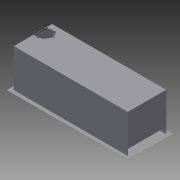
# Autodesk Inventor part: Restivo_Drawing
Saved by Autodesk Inventor 2013 SP2 (Build 170200200, 200)
## iProperties
Created: 2014-01-21
Part Number: Restivo_Drawing
Material: Generic
Document SubType Name: Modeling
Designer: mcgratta
Density: 1 g/cm^3
Author: mcgratta
Autodesk Inventor part; units mm, degrees
ref_plane "YZ Plane" through (0, 0, 0) normal (1, 0, 0) x (0, 1, 0)
ref_plane "XZ Plane" through (0, 0, 0) normal (0, 1, 0) x (-1, 0, 0)
ref_plane "XY Plane" through (0, 0, 0) normal (0, 0, 1) x (1, 0, 0)
sketch "Sketch1" plane through (0, 0, 0) normal (0, 1, 0) x (-1, 0, 0)
  line L0 (300, 300) -> (-9300, 300)
  line L1 (-9300, 300) -> (-9300, -3300)
  line L2 (-9300, -3300) -> (300, -3300)
  line L3 (300, -3300) -> (300, 300)
  point P0 (0, 0)
  dimension "d0" = 3600
  dimension "d2" = 9600
  dimension "d3" = 300
  dimension "d4" = 300
  constraints: 8 end point, 2 parallel, 1 horizontal, 1 perpendicular
  measures "d0" distance of L2.end L0.start
  measures "d2" distance between parallel lines of L1 L3
  measures "d3" distance from line of point (0, 0) L3
  measures "d4" distance from line of point (0, 0) L0
extrude "Extrusion1" add sketch "Sketch1" along normal blind 10
sketch "Sketch2" plane through (0, 10, 0) normal (0, 1, 0) x (1, 0, 0)
  line L0 (0, 0) -> (9000, 0)
  line L1 (9000, 0) -> (9000, 3000)
  line L2 (9000, 3000) -> (0, 3000)
  line L3 (0, 3000) -> (0, 0)
  line L4 (-20, -20) -> (9020, -20)
  line L5 (9020, -20) -> (9020, 3020)
  line L6 (9020, 3020) -> (-20, 3020)
  line L7 (-20, 3020) -> (-20, -20)
  dimension "d7" = 9000
  dimension "d9" = 3000
  dimension "d10" = 20
  dimension "d11" = 20
  dimension "d12" = 20
  dimension "d13" = 20
  constraints: 16 end point, 4 parallel, 2 horizontal, 2 perpendicular
  measures "d7" distance between parallel lines of L1 L3
  measures "d9" distance between parallel lines of L0 L2
  measures "d10" distance between parallel lines of L3 L7
  measures "d11" distance between parallel lines of L2 L6
  measures "d12" distance between parallel lines of L0 L4
  measures "d13" distance between parallel lines of L1 L5
extrude "Extrusion2" add sketch "Sketch2" along normal blind 3000
sketch "Sketch3" plane through (9020, 10, 20) normal (1, 0, 0) x (0, 0, -1)
  line L0 (0, 3000) -> (3040, 3000)
  line L1 (3040, 3000) -> (3040, 3020)
  line L2 (3040, 3020) -> (0, 3020)
  line L3 (0, 3020) -> (0, 3000)
  point P0 (20, -10)
  dimension "d16" = 20
  constraints: 8 end point, 2 parallel, 1 horizontal, 1 perpendicular
  measures "d16" distance between parallel lines of L0 L2
extrude "Extrusion3" add sketch "Sketch3" against normal blind 9040
sketch "Sketch4" plane through (9020, 10, 20) normal (1, 0, 0) x (0, 0, -1)
  line L0 (3040, 0) -> (0, 0) projected
  line L1 (0, 0) -> (0, 3020) projected
  line L2 (20, 0) -> (3020, 0)
  line L3 (3020, 0) -> (3020, 480)
  line L4 (3020, 480) -> (20, 480)
  line L5 (20, 480) -> (20, 0)
  point P0 (20, -10)
  dimension "d20" = 20
  dimension "d21" = 480
  dimension "d22" = 3000
  constraints: 8 end point, 2 parallel, 1 horizontal, 1 perpendicular, 1 point on line
  measures "d20" distance between parallel lines of L5 L1
  measures "d21" distance between parallel lines of L4 L0
  measures "d22" distance between parallel lines of L3 L5
extrude "Extrusion4" cut sketch "Sketch4" along normal mid plane 40
sketch "Sketch5" plane through (-20, 10, -3020) normal (-1, 0, 0) x (0, 0, 1)
  line L0 (3040, 3020) -> (0, 3020) projected
  line L1 (0, 0) -> (0, 3020) projected
  line L2 (20, 3000) -> (3020, 3000)
  line L3 (3020, 3000) -> (3020, 2832)
  line L4 (3020, 2832) -> (20, 2832)
  line L5 (20, 2832) -> (20, 3000)
  point P0 (3020, -10)
  dimension "d25" = 20
  dimension "d26" = 20
  dimension "d27" = 168
  dimension "d28" = 3000
  constraints: 8 end point, 2 parallel, 1 horizontal, 1 perpendicular
  measures "d25" distance between parallel lines of L5 L1
  measures "d26" distance between parallel lines of L2 L0
  measures "d27" distance between parallel lines of L4 L2
  measures "d28" distance between parallel lines of L3 L5
extrude "Extrusion5" cut sketch "Sketch5" against normal blind 40
sketch "Sketch7" plane through (9020, 3030, 20) normal (0, 1, 0) x (1, 0, 0)
  line L0 (-9040, 0) -> (-9040, 3040) projected
  line L1 (-9020, 2572.2782) -> (-8358.5458, 2666.2061)
  line L2 (-8358.5458, 2666.2061) -> (-8050.671, 2186.1301)
  line L3 (-8050.671, 2186.1301) -> (-8358.5458, 1669.5265)
  line L4 (-8358.5458, 1669.5265) -> (-8749.9121, 1520)
  line L5 (-8749.9121, 1520) -> (-9020, 1594.7633)
  line L6 (-9020, 1594.7633) -> (-9020, 2572.2782)
  point P0 (-9020, 20)
  constraints: 12 end point, 1 parallel
extrude "Extrusion7" cut sketch "Sketch7" against normal blind 40
body "Solid1"
